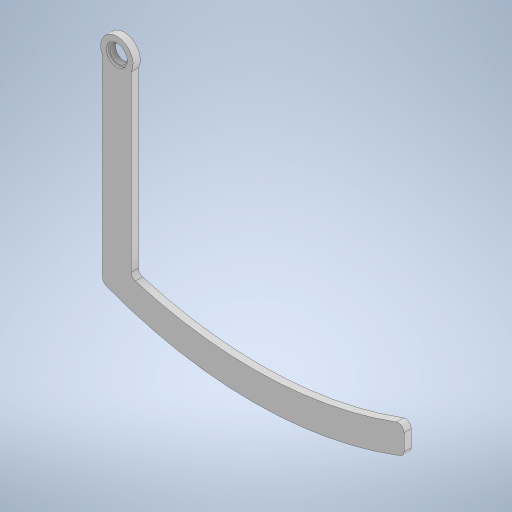
# Autodesk Inventor part: 指_大
Saved by Autodesk Inventor 2024.3 (Build 283343000, 343)
## iProperties
Created: 2024-10-09
Part Number: 指_大
Material: 一般
Document SubType Name: Modeling
Designer: hikou
Density: 1 g/cm^3
Appearance: 既定
Author: hikou
Autodesk Inventor part; units mm, degrees
ref_plane "YZ Plane" through (0, 0, 0) normal (1, 0, 0) x (0, 1, 0)
ref_plane "XZ Plane" through (0, 0, 0) normal (0, 1, 0) x (-1, 0, 0)
ref_plane "XY Plane" through (0, 0, 0) normal (0, 0, 1) x (1, 0, 0)
sketch "スケッチ1" plane through (0, 0, 0) normal (0, 0, 1) x (1, 0, 0)
  line L0 (-5, -38) -> (5, -38)
  line L1 (5, -38) -> (5, 38)
  line L2 (5, 38) -> (-5, 38)
  line L3 (-5, 38) -> (-5, -38)
  line L4 (-5, -38) -> (5, 38) construction
  line L5 (5, -38) -> (-5, 38) construction
  line L6 (-5, -38) -> (100, -38)
  line L7 (100, -38) -> (100, -28)
  line L8 (100, -28) -> (-5, -28)
  line L9 (-5, -28) -> (-5, -38)
  line L10 (47.5, -38) -> (47.5, -48)
  arc A0 (-5, -28) -> (100, -28) centre (47.5, 104.8125) ccw
  arc A1 (-5, -38) -> (100, -38) centre (47.5, 94.8125) ccw
  point P0 (0, 0)
  point P1 (5, -31.5296)
  dimension "d0" = 10
  dimension "d1" = 76
  dimension "d2" = 105
  dimension "d3" = 10
  dimension "d4" = 10
  constraints: 22 end point, 6 point on circle, 4 parallel, 3 midpoint, 2 centre point, 2 horizontal, 2 perpendicular, 1 vertical
  measures "d0" distance of L2.end L1.end
  measures "d1" distance of L0.end L1.end
  measures "d2" distance of L8.end L7.end
  measures "d3" distance of L6.end L7.end
  measures "d4" distance of L10.start L10.end
extrude "押し出し1" add sketch "スケッチ1" along normal mid plane 2.5 contours L3 A0 L1 L0 | L0 L6 L10 A1 | L1 A0 L6 | L3 L2 L1 L8 | L8 L1 A0 | L10 L6 A1 | A0 L7 L6 picked at (-0.5654, -28.4196)
sketch "スケッチ2" plane through (0, 0, 1.25) normal (0, 0, 1) x (1, 0, 0)
  line L0 (5, 38) -> (-5, 38) projected
  line L1 (5, -31.5296) -> (5, 38) projected
  circle A0 centre (0, 33) radius 3.05
  circle A1 centre (0, 33) radius 3.65
  point P0 (0, 0)
  dimension "d7" = 5
  dimension "d8" = 5
  dimension "d9" = 6.1
  dimension "d10" = 7.3
  constraints: 2 centre point, 2 coincident
  measures "d7" distance from line of L0 point (0, 33)
  measures "d8" distance from line of L1 point (0, 33)
  measures "d9" diameter of A0
  measures "d10" diameter of A1
extrude "押し出し2" cut sketch "スケッチ2" against normal blind 0.6 contours A0 | A1
sketch "スケッチ3" plane through (0, 33, 0.65) normal (0, 0, 1) x (1, 0, 0)
  circle A0 centre (0, 0) radius 3.05
  point P0 (0, -33)
  dimension "d13" = 6.1
  constraints: 1 centre point
  measures "d13" diameter of A0
extrude "押し出し3" cut sketch "スケッチ3" against normal blind 1.9
sketch "スケッチ6" plane through (0, 0, 1.25) normal (0, 0, 1) x (1, 0, 0)
  circle A0 centre (0, 33) radius 3.65 projected
  line L0 (-5, 38) -> (-5, -38) projected
  arc A1 (-5, -38) -> (100, -38) centre (47.5, 94.8125) ccw projected
  line L1 (100, -38) -> (100, -28) projected
  arc A2 (5, -31.5296) -> (100, -28) centre (47.5, 104.8125) ccw projected
  line L2 (5, -31.5296) -> (5, 38) projected
  line L3 (5, 38) -> (-5, 38) projected
  circle A3 centre (0, 33) radius 5.65
  point P0 (0, 0)
  point P1 (-5, 30.3689)
  point P2 (-5, 35.6311)
  point P3 (-2.6311, 38)
  point P4 (2.6311, 38)
  point P5 (5, 35.6311)
  point P6 (5, 30.3689)
  dimension "d18" = 11.3
  constraints: 1 centre point, 1 coincident
  measures "d18" diameter of A3
extrude "押し出し5" add sketch "スケッチ6" against normal blind 2.5 contours L0 A3 | A3 L3 | L2 A3
sketch "スケッチ7" plane through (0, 0, 1.25) normal (0, 0, 1) x (1, 0, 0)
  circle A0 centre (0, 33) radius 3.65 projected
  line L0 (-5, 38) -> (-5, 35.6311) projected
  arc A1 (-5, 35.6311) -> (-5, 30.3689) centre (0, 33) ccw projected
  line L1 (-5, 30.3689) -> (-5, -38) projected
  arc A2 (-5, -38) -> (100, -38) centre (47.5, 94.8125) ccw projected
  line L2 (100, -38) -> (100, -28) projected
  arc A3 (5, -31.5296) -> (100, -28) centre (47.5, 104.8125) ccw projected
  line L3 (5, -31.5296) -> (5, 30.3689) projected
  arc A4 (5, 30.3689) -> (5, 35.6311) centre (0, 33) ccw projected
  line L4 (5, 35.6311) -> (5, 38) projected
  line L5 (5, 38) -> (2.6311, 38) projected
  arc A5 (2.6311, 38) -> (-2.6311, 38) centre (0, 33) ccw projected
  line L6 (-2.6311, 38) -> (-5, 38) projected
  circle A6 centre (0, 33) radius 5.65
  point P0 (0, 0)
  point P1 (-5, 35.6311)
  point P2 (-2.6311, 38)
  point P3 (2.6311, 38)
  point P4 (5, 35.6311)
  constraints: 1 centre point, 1 coincident
extrude "押し出し6" cut sketch "スケッチ7" against normal blind 2.5 contours L6 A6 L0 | L5 L4 A6
fillet "フィレット1" radius 2 4 edges at (-5, -38, 0) (5, -31.5296, 0) (100, -28, 0) (100, -38, 0)
